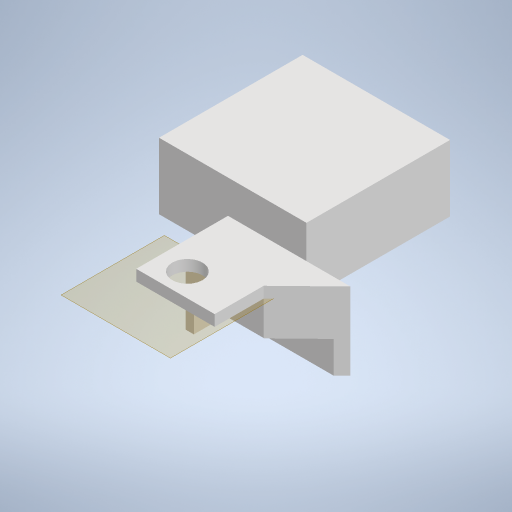
# Autodesk Inventor part: каретка
Saved by Autodesk Inventor 2024.2 (Build 282272000, 272)
## iProperties
Created: 2026-02-13
Part Number: каретка
Material: Типовые
Document SubType Name: Modeling
Designer: Service
Density: 1 g/cm^3
Appearance: По умолчанию
Author: Service
Autodesk Inventor part; units mm, degrees
ref_plane "YZ Plane" through (0, 0, 0) normal (1, 0, 0) x (0, 1, 0)
ref_plane "XZ Plane" through (0, 0, 0) normal (0, 1, 0) x (-1, 0, 0)
ref_plane "XY Plane" through (0, 0, 0) normal (0, 0, 1) x (1, 0, 0)
ref_plane "РабПлоскость1" through (-7.5749, -280.0826, 223.3085) normal (0, 1, 0) x (-1, 0, 0)
sketch "Эскиз1" plane through (-7.5749, -280.0826, 223.3085) normal (0, 1, 0) x (-1, 0, 0)
  line L0 (14.2093, 2.6473) -> (0, 2.6473)
  line L1 (0, 2.6473) -> (0, -6.2943)
  line L2 (0, -6.2943) -> (14.2093, -6.2943)
  line L3 (14.2093, -6.2943) -> (14.2093, 2.6473)
  line L4 (4.1714, -6.2943) -> (16.1714, -6.2943) projected
  line L5 (0, -6.2943) -> (0, -6.2338) projected
  circle A0 centre (9.1714, -1.5852) radius 2.75 projected
  line L6 (0, -6.2338) -> (-7.9567, -13.9803)
  line L7 (-7.9567, -13.9803) -> (14.2093, -13.9803)
  line L8 (14.2093, -13.9803) -> (14.2093, -6.2943)
  line L9 (-6.416, -12.4803) -> (14.2093, -12.4803)
  line L10 (12.7093, -6.2943) -> (12.7093, -12.4803)
  point P0 (-7.5749, -223.3085)
  point P1 (6.5045, -0.9144)
  point P2 (6.5045, -2.256)
  point P3 (0, -6.2338)
  point P4 (12.7093, -6.2943)
  dimension "d2" = 1.5
  dimension "d3" = 1.5
  constraints: 18 end point, 4 perpendicular, 4 point on line, 2 collinear, 2 horizontal, 2 parallel
  measures "d2" distance between parallel lines of L8 L10
  measures "d3" distance between parallel lines of L9 L7
extrude "Выдавливание1" add sketch "Эскиз1" along normal blind 2
extrude "Выдавливание2" add sketch "Эскиз1" against normal blind 12 contours L8 L9 L10 L2 | L8 L7 L6 L9
extrude "Выдавливание3" add sketch "Эскиз1" against normal blind 6.25 contours L1 L2 L10 L9 L6
sketch "Эскиз2" plane through (-7.5749, -278.0826, 223.3085) normal (0, 1, 0) x (1, 0, 0)
  line L0 (-14.2093, 13.9803) -> (7.9567, 13.9803) projected
  line L1 (0.0011, 13.9803) -> (-26.6989, 13.9803)
  line L2 (-26.6989, 13.9803) -> (-26.6989, 39.9803)
  line L3 (-26.6989, 39.9803) -> (0.0011, 39.9803)
  line L4 (0.0011, 39.9803) -> (0.0011, 13.9803)
  point P0 (7.5749, 223.3085)
  point P1 (-14.2093, 6.2943)
  dimension "d9" = 26
  dimension "d10" = 26.7
  constraints: 8 end point, 2 parallel, 1 horizontal, 1 perpendicular, 1 point on line
  measures "d9" distance of L3.end L1.start
  measures "d10" distance of L2.end L3.end
extrude "Выдавливание4" add sketch "Эскиз2" along normal mid plane 12
